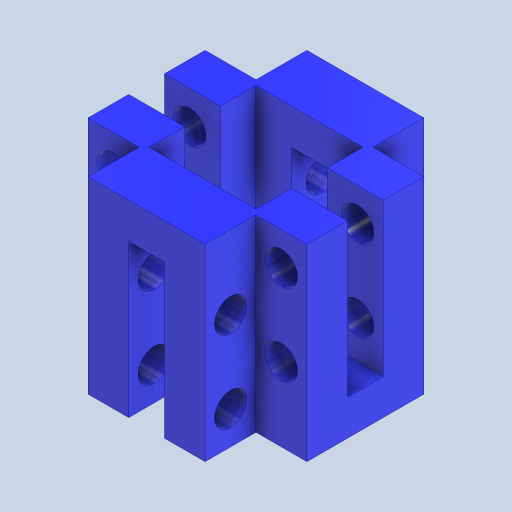
# Autodesk Inventor part: RZvector-Srunit-v2-3DP-Spacer
Saved by Autodesk Inventor 2024 (Build 280153000, 153)
## iProperties
Created: 2024-04-13
Part Number: RZvector-Srunit-v2-3DP-Spacer
Material: ABS プラスチック
Document SubType Name: Modeling
Designer: haruy
Density: 1.06 g/cm^3
Appearance: 青 - 壁塗料 - 光沢
Author: haruy
Autodesk Inventor part; units mm, degrees
ref_plane "YZ Plane" through (0, 0, 0) normal (1, 0, 0) x (0, 1, 0)
derived "RZvector-Srunit-v2-Sketch-Base.ipt"
sketch "正面から" plane through (0, 0, 0) normal (0, 0, 1) x (1, 0, 0)
  line L0 (0, 0) -> (20, 0)
  line L1 (20, 0) -> (20, 80)
  line L2 (20, 80) -> (0, 80)
  line L3 (0, 80) -> (0, 0)
  line L4 (21.5, 92) -> (31.5, 92)
  line L5 (31.5, 92) -> (31.5, 0)
  line L6 (31.5, 0) -> (21.5, 0)
  line L7 (21.5, 0) -> (21.5, 92)
  line L8 (-11.5, 62) -> (-1.5, 62)
  line L9 (-1.5, 62) -> (-1.5, 0)
  line L10 (-1.5, 0) -> (-11.5, 0)
  line L11 (-11.5, 0) -> (-11.5, 62)
  line L12 (-1.5, 24.5) -> (21.5, 24.5)
  line L13 (21.5, 24.5) -> (21.5, 18.5)
  line L14 (21.5, 18.5) -> (-1.5, 18.5)
  line L15 (-1.5, 18.5) -> (-1.5, 24.5)
  line L16 (7.5, 28) -> (12.5, 28)
  line L17 (12.5, 28) -> (12.5, 15)
  line L18 (12.5, 15) -> (7.5, 15)
  line L19 (7.5, 15) -> (7.5, 28)
  circle A0 centre (26.5, 29.5) radius 3
  line L20 (31.5, 15) -> (-189.7387, 15)
  line L21 (-189.7387, 15) -> (-189.7387, 0)
  line L22 (-189.7387, 0) -> (31.5, 0)
  line L23 (31.5, 0) -> (31.5, 15)
  line L24 (31.5, 92) -> (41.5, 92)
  line L25 (41.5, 92) -> (41.5, 62)
  line L26 (41.5, 62) -> (31.5, 62)
  line L27 (31.5, 62) -> (31.5, 92)
  circle A1 centre (26.5, 29.5) radius 6.5
  circle A2 centre (-6.5, 29.5) radius 6.5
  line L28 (21.5, 23) -> (31.5, 23)
  line L29 (21.5, 20) -> (31.5, 20)
  circle A3 centre (26.5, 29.5) radius 1.5
  circle A4 centre (-6.5, 29.5) radius 3
  circle A5 centre (-6.5, 29.5) radius 1.5
  line L30 (-1.5, 40.5) -> (21.5, 40.5)
  line L31 (21.5, 40.5) -> (21.5, 34.5)
  line L32 (21.5, 34.5) -> (-1.5, 34.5)
  line L33 (-1.5, 34.5) -> (-1.5, 40.5)
  line L34 (7.5, 44) -> (12.5, 44)
  line L35 (12.5, 44) -> (12.5, 31)
  line L36 (12.5, 31) -> (7.5, 31)
  line L37 (7.5, 31) -> (7.5, 44)
  circle A6 centre (-6.5, 45.5) radius 6.5
  circle A7 centre (-6.5, 45.5) radius 3
  circle A8 centre (-6.5, 45.5) radius 1.5
  line L38 (-11.5, 62) -> (31.5, 62)
  line L39 (31.5, 62) -> (31.5, 52)
  line L40 (31.5, 52) -> (-11.5, 52)
  line L41 (-11.5, 52) -> (-11.5, 62)
  circle A9 centre (26.5, 45.5) radius 6.5
  circle A10 centre (26.5, 45.5) radius 3
  circle A11 centre (26.5, 45.5) radius 1.5
  line L42 (6.5, 15) -> (6.5, 30)
  line L43 (6.5, 30) -> (13.5, 30)
  line L44 (13.5, 30) -> (13.5, 15)
  line L45 (13.5, 45) -> (6.5, 45)
  line L46 (6.5, 45) -> (6.5, 30)
  line L47 (6.5, 30) -> (13.5, 30)
  line L48 (13.5, 30) -> (13.5, 45)
  point P0 (-1.5, 15)
  point P1 (21.5, 15)
  point P2 (21.5, 52)
  point P3 (-1.5, 52)
  dimension "d2" = 1
  dimension "d3" = 1
  dimension "d4" = 2
  dimension "d5" = 1
  measures "d2" distance between parallel lines of L42 L19
  measures "d3" distance between parallel lines of L17 L44
  measures "d4" distance between parallel lines of L16 L43
  measures "d5" distance between parallel lines of L34 L45
sketch "横から" plane through (0, 0, 0) normal (1, 0, 0) x (0, 1, 0)
  line L0 (0, 0) -> (200, 0)
  line L1 (200, 0) -> (200, -20)
  line L2 (200, -20) -> (0, -20)
  line L3 (0, -20) -> (0, 0)
  circle A0 centre (21.5, 6.5) radius 6.5
  circle A1 centre (21.5, -26.5) radius 6.5
  line L4 (15, 26.5) -> (0, 26.5)
  line L5 (0, 26.5) -> (0, 11.5)
  line L6 (0, 11.5) -> (15, 11.5)
  line L7 (15, 11.5) -> (15, 26.5)
  line L8 (15, -31.5) -> (0, -31.5)
  line L9 (0, -31.5) -> (0, -46.5)
  line L10 (0, -46.5) -> (15, -46.5)
  line L11 (15, -46.5) -> (15, -31.5)
  line L12 (62, 11.5) -> (0, 11.5)
  line L13 (0, 11.5) -> (0, 1.5)
  line L14 (0, 1.5) -> (62, 1.5)
  line L15 (62, 1.5) -> (62, 11.5)
  line L16 (62, -21.5) -> (0, -21.5)
  line L17 (0, -21.5) -> (0, -31.5)
  line L18 (0, -31.5) -> (62, -31.5)
  line L19 (62, -31.5) -> (62, -21.5)
  line L20 (36, -7.5) -> (23, -7.5)
  line L21 (23, -7.5) -> (23, -12.5)
  line L22 (23, -12.5) -> (36, -12.5)
  line L23 (36, -12.5) -> (36, -7.5)
  line L24 (92, 11.5) -> (62, 11.5)
  line L25 (62, 11.5) -> (62, -31.5)
  line L26 (62, -31.5) -> (92, -31.5)
  line L27 (92, -31.5) -> (92, 11.5)
  circle A2 centre (37.5, 6.5) radius 6.5
  circle A3 centre (37.5, -26.5) radius 6.5
  line L28 (52, -7.5) -> (39, -7.5)
  line L29 (39, -7.5) -> (39, -12.5)
  line L30 (39, -12.5) -> (52, -12.5)
  line L31 (52, -12.5) -> (52, -7.5)
  point P0 (62, -26.5)
extrude "押し出し1" add sketch "正面から" along normal blind 10 contours L20 L9 L14 L3 | L3 L14 L42 L20 | L20 L44 L14 L1 | L1 L14 L7 L20 | L14 L9 L12 L3 | L3 L12 L42 L14 | L14 L44 L12 L1 | L1 L12 L7 L14 | L12 L9 A2 L3 | L3 L32 L46 L42 L12 | L12 L44 L48 L32 L1 | L1 A1 L7 L12 | A2 L9 L32 L3 | A2 L9 | L1 L32 L7 A1 | A1 L7 | L32 L9 L30 L3 | L3 L30 L46 L32 | L32 L48 L30 L1 | L1 L30 L7 L32 | L30 L9 A6 L3 | L3 L40 L1 L30 L48 L45 L46 | L1 A9 L7 L30 | A6 L9 L40 L3 | A6 L9 | L1 L40 L7 A9 | A9 L7
ref_plane "作業平面1" through (21.5, 52, -11.5) normal (0, 0, -1) x (-1, 0, 0)
mirror "ミラー1" about plane through (21.5, 52, -11.5) normal (0, 0, -1) of "押し出し1"
sketch "スケッチ4" plane through (21.5, 15, 0) normal (1, 0, 0) x (0, 0, -1)
  line L0 (9, 21) -> (14, 21)
  line L1 (14, 21) -> (14, 8)
  line L2 (14, 8) -> (9, 8)
  line L3 (9, 8) -> (9, 21)
  line L4 (9, 37) -> (14, 37)
  line L5 (14, 37) -> (14, 24)
  line L6 (14, 24) -> (9, 24)
  line L7 (9, 24) -> (9, 37)
  line L8 (23, 37) -> (33, 37) projected
  line L9 (23, 0) -> (23, 37) projected
  line L10 (0, 37) -> (0, 0) projected
  line L11 (0, 37) -> (23, 37)
  line L12 (23, 37) -> (23, 0)
  line L13 (23, 0) -> (0, 0)
  line L14 (0, 0) -> (0, 37)
  line L15 (15, 22) -> (8, 22)
  line L16 (8, 22) -> (8, 7)
  line L17 (8, 7) -> (15, 7)
  line L18 (15, 7) -> (15, 22)
  line L19 (8, 37) -> (8, 22)
  line L20 (8, 22) -> (15, 22)
  line L21 (15, 22) -> (15, 37)
  point P0 (0, -15)
  point P1 (0, 0)
  dimension "d9" = 5
  dimension "d10" = 13
  dimension "d11" = 5
  dimension "d12" = 13
  dimension "d13" = 0
  dimension "d14" = 9
  dimension "d15" = 9
  dimension "d16" = 3
  dimension "d17" = 1
  dimension "d18" = 1
  dimension "d19" = 2
  dimension "d20" = 1
  constraints: 38 end point, 8 parallel, 6 perpendicular, 3 horizontal, 2 point on line, 1 vertical, 3 other
  measures "d9" distance of L1.end L2.end
  measures "d10" distance of L0.end L1.end
  measures "d11" distance of L5.end L6.end
  measures "d12" distance of L4.end L5.end
  measures "d13" distance between parallel lines of L4 L8
  measures "d14" distance between parallel lines of L5 L9
  measures "d15" distance between parallel lines of L1 L9
  measures "d16" distance between parallel lines of L6 L0
  measures "d17" distance between parallel lines of L0 L15
  measures "d18" distance between parallel lines of L19 L7
  measures "d19" distance between parallel lines of L20 L6
  measures "d20" distance between parallel lines of L21 L5
extrude "押し出し2" add sketch "スケッチ4" along normal blind 10 contours L19 L16 L17 L18 L21 L11 L9 L13 L10
ref_plane "作業平面2" through (10, 15, 0) normal (-1, 0, 0) x (0, 0, 1)
mirror "ミラー2" about plane through (10, 15, 0) normal (-1, 0, 0) of "押し出し2"
sketch "スケッチ5" plane through (-1.5, 15, 0) normal (0, 0, 1) x (1, 0, 0)
  line L0 (0, 37) -> (-10, 37) projected
  line L1 (-10, 37) -> (-10, 0) projected
  line L2 (33, 37) -> (33, 0) projected
  line L3 (23, 37) -> (33, 37) projected
  point P0 (1.5, -15)
  point P1 (-5, 30.5)
  point P2 (-5, 14.5)
  point P3 (28, 30.5)
  point P4 (28, 14.5)
  dimension "d25" = 6.5
  dimension "d26" = 5
  dimension "d27" = 16
  dimension "d28" = 5
  dimension "d29" = 5
  dimension "d30" = 6.5
  dimension "d31" = 16
  dimension "d32" = 5
  measures "d25" distance from line of point (-5, 30.5) L0
  measures "d26" distance from line of L1 point (-5, 30.5)
  measures "d27" distance of point (-5, 14.5) point (-5, 30.5)
  measures "d28" distance from line of point (-5, 14.5) L1
  measures "d29" distance from line of L2 point (28, 30.5)
  measures "d30" distance from line of point (28, 30.5) L3
  measures "d31" distance of point (28, 14.5) point (28, 30.5)
  measures "d32" distance from line of point (28, 14.5) L2
hole "穴1" at (-6.5, 45.5, 0) at (-6.5, 29.5, 0) at (26.5, 45.5, 0) at (26.5, 29.5, 0) direction (0, 0, -1) diameter 6.3 end through all
sketch "スケッチ6" plane through (21.5, 15, 10) normal (1, 0, 0) x (0, 0, -1)
  line L0 (0, 0) -> (0, 37) projected
  line L1 (10, 0) -> (0, 0) projected
  line L2 (43, 0) -> (43, 37) projected
  line L3 (33, 0) -> (43, 0) projected
  point P0 (10, -15)
  point P1 (5, 6.5)
  point P2 (5, 22.5)
  point P3 (38, 22.5)
  point P4 (38, 6.5)
  dimension "d40" = 5
  dimension "d41" = 5
  dimension "d42" = 6.5
  dimension "d43" = 16
  dimension "d44" = 5
  dimension "d45" = 5
  dimension "d46" = 6.5
  dimension "d47" = 16
  measures "d40" distance from line of L0 point (5, 6.5)
  measures "d41" distance from line of L0 point (5, 22.5)
  measures "d42" distance from line of point (5, 6.5) L1
  measures "d43" distance of point (5, 22.5) point (5, 6.5)
  measures "d44" distance from line of L2 point (38, 6.5)
  measures "d45" distance from line of point (38, 22.5) L2
  measures "d46" distance from line of point (38, 6.5) L3
  measures "d47" distance of point (38, 22.5) point (38, 6.5)
hole "穴2" at (21.5, 21.5, 5) at (21.5, 37.5, 5) at (21.5, 37.5, -28) at (21.5, 21.5, -28) direction (-1, 0, 0) diameter 6.3 end through all
sketch "スケッチ7" plane through (-1.5, 52, -33) normal (0, 1, 0) x (1, 0, 0)
  line L0 (1.5, -31.5) -> (21.5, -31.5)
  line L1 (21.5, -31.5) -> (21.5, -11.5)
  line L2 (21.5, -11.5) -> (1.5, -11.5)
  line L3 (1.5, -11.5) -> (1.5, -31.5)
  line L4 (23, -10) -> (0, -10) projected
  line L5 (0, -10) -> (0, -18) projected
  line L6 (1, -11) -> (22, -11)
  line L7 (22, -11) -> (22, -32)
  line L8 (22, -32) -> (1, -32)
  line L9 (1, -32) -> (1, -11)
  line L10 (23, -25) -> (23, -33) projected
  line L11 (0, -10) -> (23, -10)
  line L12 (23, -10) -> (23, -33)
  line L13 (23, -33) -> (0, -33)
  line L14 (0, -33) -> (0, -10)
  point P0 (1.5, -33)
  dimension "d55" = 20
  dimension "d56" = 20
  dimension "d57" = 1.5
  dimension "d58" = 1.5
  dimension "d59" = 0.5
  constraints: 24 end point, 6 parallel, 3 perpendicular, 2 horizontal, 3 other
  measures "d55" distance of L2.end L1.end
  measures "d56" distance of L2.end L0.start
  measures "d57" distance between parallel lines of L2 L4
  measures "d58" distance between parallel lines of L5 L3
  measures "d59" distance between parallel lines of L2 L6
extrude "押し出し3" add sketch "スケッチ7" against normal up to surface (37 mm away) contours L12 L10 L13 L14 L5 L4
sketch "スケッチ8" plane through (-1.5, 52, 10) normal (0, 0, 1) x (1, 0, 0)
  line L0 (8, -7) -> (15, -7) projected
  line L1 (15, -7) -> (15, -22) projected
  line L2 (8, -7) -> (15, -7)
  line L3 (15, -7) -> (15, -22)
  line L4 (15, -22) -> (8, -22)
  line L5 (8, -22) -> (8, -7)
  line L6 (15, -37) -> (8, -37) projected
  line L7 (8, -23) -> (15, -23) projected
  line L8 (15, -37) -> (8, -37)
  line L9 (8, -37) -> (8, -23)
  line L10 (8, -23) -> (15, -23)
  line L11 (15, -23) -> (15, -37)
  line L12 (8, -23) -> (15, -23)
  line L13 (15, -23) -> (15, -22)
  line L14 (15, -22) -> (8, -22)
  line L15 (8, -22) -> (8, -23)
  point P0 (1.5, -52)
  constraints: 24 end point, 6 parallel, 3 horizontal, 3 perpendicular
extrude "押し出し4" cut sketch "スケッチ8" against normal through all
sketch "スケッチ9" plane through (31.5, 15, 0) normal (1, 0, 0) x (0, 0, -1)
  line L0 (15, 37) -> (8, 37) projected
  line L1 (14.5, 37) -> (14.5, 23.5) projected
  line L2 (8, 37) -> (14.5, 37)
  line L3 (14.5, 37) -> (14.5, 23.5)
  line L4 (14.5, 23.5) -> (8, 23.5)
  line L5 (8, 23.5) -> (8, 37)
  line L6 (8.5, 7) -> (8.5, 21.5) projected
  line L7 (15, 7) -> (8, 7) projected
  line L8 (8.5, 21.5) -> (15, 21.5)
  line L9 (15, 21.5) -> (15, 7)
  line L10 (15, 7) -> (8.5, 7)
  line L11 (8.5, 7) -> (8.5, 21.5)
  line L12 (15, 7) -> (8, 7)
  line L13 (8, 7) -> (8, 23.5)
  line L14 (8, 23.5) -> (15, 23.5)
  line L15 (15, 23.5) -> (15, 7)
  line L16 (8, 37) -> (15, 37)
  line L17 (15, 37) -> (15, 23.5)
  line L18 (15, 23.5) -> (8, 23.5)
  line L19 (8, 23.5) -> (8, 37)
  point P0 (0, -15)
  constraints: 32 end point, 8 parallel, 4 horizontal, 4 perpendicular, 2 other
extrude "押し出し5" cut sketch "スケッチ9" against normal through all
equation "\"d28\" = d26"
equation "\"d32\" = d29"
equation "\"d41\" = d40"
equation "\"d44\" = d40"
equation "\"d45\" = d40"
equation "\"d46\" = d42"
equation "\"d47\" = d43"
